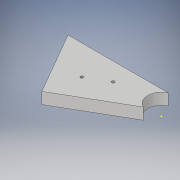
# Autodesk Inventor part: flipper-hug-left-2
Saved by Autodesk Inventor 2017 (Build 210142000, 142)
## iProperties
Created: 2017-02-21
Part Number: flipper-hug-left-2
Material: Generic
Document SubType Name: Modeling
Designer: John
Density: 1 g/cm^3
Appearance: Default
Author: John
Autodesk Inventor part; units mm, degrees
ref_plane "YZ Plane" through (0, 0, 0) normal (1, 0, 0) x (0, 1, 0)
ref_plane "XZ Plane" through (0, 0, 0) normal (0, 1, 0) x (-1, 0, 0)
ref_plane "XY Plane" through (0, 0, 0) normal (0, 0, 1) x (1, 0, 0)
sketch "Sketch1" plane through (0, 0, 0) normal (0, 1, 0) x (-1, 0, 0)
  point P0 (0, 0)
sketch "Sketch2" plane through (0, 0, 0) normal (0, 1, 0) x (-1, 0, 0)
  circle A0 centre (0, 0) radius 10 construction
  arc A1 (5.0714, -10.8757) -> (5.0714, 10.8757) centre (0, 0) ccw
  line L0 (5.0714, 10.8757) -> (5.0714, -10.8757) construction
  line L1 (5.0714, -10.8757) -> (92.8296, -10.8757)
  line L2 (5.0714, -10.8757) -> (92.8296, -10.8757) construction
  line L3 (80.2714, 10.8757) -> (92.8296, -10.8757)
  line L4 (80.2714, 10.8757) -> (5.0714, 10.8757)
  dimension "d0" = 20
  dimension "d2" = 2
  dimension "d3" = 130
  dimension "d5" = 0
  dimension "d14" = 75.2
  dimension "d15" = 12.5582
  constraints: 10 end point, 3 horizontal, 2 centre point, 2 point on circle, 1 coincident, 1 collinear, 1 concentric
  measures "d0" diameter of A0
  measures "d2" radial gap between concentric circles of A1 A0
  measures "d5" distance between parallel lines of L1 L2
  measures "d14" distance of L3.start L0.start
  measures "d15" horizontal distance of L3.start L2.end
extrude "Extrusion1" add sketch "Sketch2" along normal blind 10
sketch "Sketch3" plane through (0, 10, 0) normal (0, 1, 0) x (1, 0, 0)
  line L0 (-80.2714, -10.8757) -> (-92.8296, 10.8757) projected
  line L1 (-80.2714, -10.8757) -> (-61.4714, -43.4382)
  arc A0 (-5.0714, 10.8757) -> (-5.0714, -10.8757) centre (0, 0) ccw projected
  line L2 (-61.4714, -43.4382) -> (-5.0714, -10.8757)
  line L3 (-80.2714, -10.8757) -> (-5.0714, -10.8757) projected
  line L4 (-80.2714, -10.8757) -> (-5.0714, -10.8757)
  point P0 (-104.4015, 68.9975)
  point P1 (-92.8296, 10.8757)
  constraints: 6 end point, 1 horizontal, 1 perpendicular, 2 other
extrude "Extrusion2" add sketch "Sketch3" against normal blind 10
sketch "Sketch4" plane through (0, 10, 0) normal (0, 1, 0) x (1, 0, 0)
  circle A0 centre (-54.7759, -15.0352) radius 1.25
  circle A1 centre (-37.4554, -5.0352) radius 1.25
  line L0 (-54.7759, -15.0352) -> (-37.4554, -5.0352) construction
  line L1 (-61.4714, -43.4382) -> (-5.0714, -10.8757) construction
  line L2 (-92.8296, 10.8757) -> (-61.4714, -43.4382) construction
  point P0 (0, 0)
  dimension "d16" = 2.5
  dimension "d17" = 2.5
  dimension "d18" = 20
  dimension "d19" = 20
  dimension "d20" = 21.25
  constraints: 2 centre point, 2 end point, 1 parallel
  measures "d16" diameter of A0
  measures "d17" diameter of A1
  measures "d18" distance of L0.start L0.end
  measures "d19" distance from line of L2 L0.start
  measures "d20" distance from line of L1 L0.start
extrude "Extrusion3" cut sketch "Sketch4" along normal through all both and the other way through all
body "Solid1"
